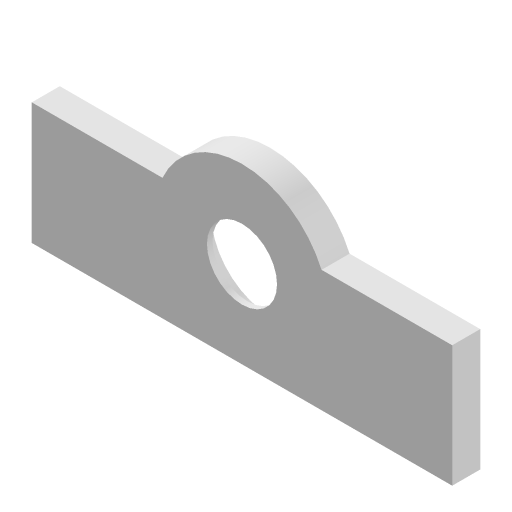
# Autodesk Inventor part: AOPORTE DE CAJA SEPARADORA
Saved by Autodesk Inventor 2024 (Build 280153000, 153)
## iProperties
Created: 2024-06-16
Part Number: AOPORTE DE CAJA SEPARADORA
Material: Generic
Document SubType Name: Modeling
Designer: Jhuliams
Density: 1 g/cm^3
Appearance: Default
Author: Jhuliams
Autodesk Inventor part; units mm, degrees
ref_plane "YZ Plane" through (0, 0, 0) normal (1, 0, 0) x (0, 1, 0)
ref_plane "XZ Plane" through (0, 0, 0) normal (0, 1, 0) x (-1, 0, 0)
ref_plane "XY Plane" through (0, 0, 0) normal (0, 0, 1) x (1, 0, 0)
sketch "Sketch1" plane through (0, 0, 0) normal (0, 0, 1) x (1, 0, 0)
  line L0 (75, 12.4416) -> (75, -12.5584)
  line L1 (75, -12.5584) -> (10.3681, -12.5584)
  line L2 (-75, -12.4416) -> (-75, 12.4948)
  line L3 (-75, 12.4948) -> (48.1392, -8.0199) construction
  line L4 (75, 12.4416) -> (-75, -12.4416) construction
  line L5 (10.3681, -12.5584) -> (111, -12.5584)
  line L6 (111, -12.5584) -> (111, -30.9416)
  line L7 (111, -30.9416) -> (-75, -30.9416)
  line L8 (-75, -30.9416) -> (-75, -12.4416)
  arc A0 (28.3798, 12.4416) -> (-28.3564, 12.4948) centre (0, 0) ccw
  circle A1 centre (0, 0) radius 12.5
  line L9 (-75, 12.4948) -> (-28.3564, 12.4948)
  line L10 (28.3798, 12.4416) -> (75, 12.4416)
  line L11 (75, -12.5584) -> (75, -30.9416)
  point P0 (93, -12.5)
  dimension "d1" = 150
  dimension "d2" = 25
  dimension "d5" = 25
  constraints: 24 end point, 5 parallel, 4 perpendicular, 3 horizontal, 2 centre point, 2 coincident, 2 point on circle, 2 point on line, 1 midpoint
  measures "d1" distance of L0.end L2.start
  measures "d2" distance of L0.start L0.end
  measures "d5" diameter of A1
extrude "Extrusion1" add sketch "Sketch1" along normal blind 10 contours L0 L11 L7 L8 L2 L9 A0 L10
sketch "Sketch2" plane through (0, 0, 0) normal (0, 0, -1) x (-1, 0, 0)
  circle A0 centre (0, 0) radius 21
  dimension "d6" = 42
  constraints: 1 centre point, 1 coincident
  measures "d6" diameter of A0
extrude "Extrusion2" cut sketch "Sketch2" against normal blind 8
body "Solid1"
